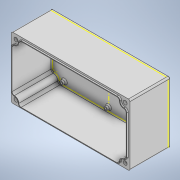
# Autodesk Inventor part: CustomBox_Rev3a
Saved by Autodesk Inventor 2021 (Build 250183000, 183)
## iProperties
Created: 2021-04-04
Part Number: CustomBox_Rev3a
Material: Generic
Document SubType Name: Modeling
Designer: James
Density: 1 g/cm^3
Appearance: Default
wall_thickness: 3.000 mm
lid_screw_d: 4.000 mm
lid_screw_offset_w: 3.182 mm
min_wall_width: 1.000 mm
inner_gasket_wall: 0.800 mm
inner_gasket_wall_h: 2.000 mm
pem_height: 4.000 mm
PEM_fillet: 1.500 mm
corner_fillet: 2.000 mm
inner_fillet: 1.000 mm
bottom_fillet: 1.000 mm
Author: James
Autodesk Inventor part; units mm, degrees
sketch "Sketch2" plane through (0, 0, 0) normal (0, 0, 1) x (1, 0, 0)
  line L0 (-78, 40.5) -> (78, 40.5)
  line L1 (78, 40.5) -> (78, -40.5)
  line L2 (78, -40.5) -> (-78, -40.5)
  line L3 (-78, -40.5) -> (-78, 40.5)
  line L4 (-78, 40.5) -> (78, -40.5) construction
  line L5 (78, 40.5) -> (-78, -40.5) construction
  line L6 (0, 40.5) -> (0, -40.5)
  line L7 (-78, 0) -> (78, 0)
  circle A0 centre (-71.818, 34.318) radius 2.5
  line L8 (-75, 29.545) -> (-67.045, 29.545) construction
  line L9 (-67.045, 29.545) -> (-67.045, 37.5) construction
  line L10 (75, 37.5) -> (-63.0835, 37.5) construction
  line L11 (-75, 25.5835) -> (-75, -37.5) construction
  line L12 (-75, -37.5) -> (75, -37.5) construction
  line L13 (75, -37.5) -> (75, 37.5) construction
  line L14 (-75, 37.5) -> (-67.045, 29.545) construction
  arc A1 (-71.9375, 28.5829) -> (-66.0829, 34.4375) centre (-71.818, 34.318) ccw
  arc A2 (-71.9375, 28.5829) -> (-75, 25.5835) centre (-72, 25.5835) ccw
  arc A3 (-63.0835, 37.5) -> (-66.0829, 34.4375) centre (-63.0835, 34.5) ccw
  line L15 (-75, 25.5835) -> (-75, 0)
  line L16 (-63.0835, 37.5) -> (0, 37.5)
  arc A4 (-66.0829, -34.4375) -> (-71.9375, -28.5829) centre (-71.818, -34.318) ccw
  arc A5 (-75, -25.5835) -> (-71.9375, -28.5829) centre (-72, -25.5835) ccw
  arc A6 (-66.0829, -34.4375) -> (-63.0835, -37.5) centre (-63.0835, -34.5) ccw
  line L17 (-75, -25.5835) -> (-75, 0)
  line L18 (-63.0835, -37.5) -> (0, -37.5)
  arc A7 (66.0829, 34.4375) -> (71.9375, 28.5829) centre (71.818, 34.318) ccw
  arc A8 (75, 25.5835) -> (71.9375, 28.5829) centre (72, 25.5835) ccw
  arc A9 (66.0829, 34.4375) -> (63.0835, 37.5) centre (63.0835, 34.5) ccw
  line L19 (75, 25.5835) -> (75, 0)
  line L20 (63.0835, 37.5) -> (0, 37.5)
  line L21 (63.0835, -37.5) -> (0, -37.5)
  arc A10 (63.0835, -37.5) -> (66.0829, -34.4375) centre (63.0835, -34.5) ccw
  arc A11 (71.9375, -28.5829) -> (66.0829, -34.4375) centre (71.818, -34.318) ccw
  arc A12 (71.9375, -28.5829) -> (75, -25.5835) centre (72, -25.5835) ccw
  line L22 (75, -25.5835) -> (75, 0)
  circle A13 centre (-71.818, -34.318) radius 2.5
  circle A14 centre (71.818, 34.318) radius 2.5
  circle A15 centre (71.818, -34.318) radius 2.5
  line L23 (0, 37.5) -> (-75, 37.5) construction
  line L24 (-75, 0) -> (-75, 37.5) construction
  point P0 (0, 0)
  point P1 (-75, 29.545)
  dimension "d5" = 156
  dimension "d6" = 81
  dimension "d11" = 5
  dimension "d23" = 3
  dimension "lid_screw_offset_w" = 3.182
  dimension "d26" = 7.955
  dimension "d27" = 7.955
  dimension "d28" = 3
  constraints: 50 end point, 26 point on circle, 26 symmetric about line, 16 centre point, 10 point on line, 6 midpoint, 4 parallel, 4 perpendicular, 4 tangent, 3 horizontal, 1 coincident, 1 equal radius, 15 other
  measures "d5" distance of L1.end L2.end
  measures "d6" distance of L0.end L1.end
  measures "d11" diameter of A0
  measures "d23" distance between parallel lines of L0 L10
  measures "lid_screw_offset_w" distance from line of A0.centre L11
  measures "d26" distance between parallel lines of L9 L11
  measures "d27" distance between parallel lines of L8 L10
  measures "d28" radius of A2
extrude "Extrusion1" add sketch "Sketch2" against normal blind 3 contours L0 L6 L16 A3 A1 A2 L15 L7 L3 | L0 L1 L7 L19 A8 A7 A9 L20 L6 | L7 L17 A5 A4 A6 L18 L6 L2 L3 | L20 A9 A7 A8 L19 L7 L6 | L6 L7 L15 A2 A1 A3 L16 | L7 L6 L18 A6 A4 A5 L17 | L1 L2 L6 L21 A10 A11 A12 L22 L7 | L7 L22 A12 A11 A10 L21 L6 | A0 | A13 | A14 | A15
extrude "Extrusion2" add sketch "Sketch2" along normal blind 50 contours L0 L6 L16 A3 A1 A2 L15 L7 L3 | L0 L1 L7 L19 A8 A7 A9 L20 L6 | L7 L17 A5 A4 A6 L18 L6 L2 L3 | L1 L2 L6 L21 A10 A11 A12 L22 L7
fillet "Fillet1" radius 2 4 edges at (-78, 40.5, 23.5) (-78, -40.5, 23.5) (78, -40.5, 23.5) (78, 40.5, 23.5)
fillet "Fillet2" radius 1 16 edges at (-65.2268, 36.5991, 0) (-67.7618, 30.2618, 0) (-74.0991, 27.7268, 0) (-75, 0, 0) (-74.0991, -27.7268, 0) (-67.7618, -30.2618, 0) (-65.2268, -36.5991, 0) (0, -37.5, 0) (65.2268, -36.5991, 0) (67.7618, -30.2618, 0) (74.0991, -27.7268, 0) (75, 0, 0) (74.0991, 27.7268, 0) (67.7618, 30.2618, 0) (65.2268, 36.5991, 0) (0, 37.5, 0)
fillet "Fillet3" radius 1 8 edges at (-77.4142, 39.9142, -3) (0, 40.5, -3) (77.4142, 39.9142, -3) (78, 0, -3) (77.4142, -39.9142, -3) (0, -40.5, -3) (-77.4142, -39.9142, -3) (-78, 0, -3)
ref_plane "Work Plane1" through (78, -40.5, 0) normal (0, 0, -1) x (-1, 0, 0)
sketch "Sketch3" plane through (78, -40.5, 0) normal (0, 0, -1) x (-1, 0, 0)
  line L0 (156, 79) -> (156, 2) projected
  line L1 (154, 0) -> (2, 0) projected
  line L2 (2, 81) -> (154, 81) projected
  line L3 (0, 2) -> (0, 79) projected
  line L4 (78, 81) -> (78, 0) projected
  line L5 (156, 40.5) -> (0, 40.5) projected
  line L6 (14.9165, 4) -> (141.0835, 4) projected
  line L7 (152, 14.9165) -> (152, 66.0835) projected
  line L8 (141.0835, 77) -> (14.9165, 77) projected
  line L9 (4, 66.0835) -> (4, 14.9165) projected
  arc A0 (12.9169, 6.0417) -> (6.0417, 12.9169) centre (6.182, 6.182) ccw projected
  arc A1 (6.0417, 68.0831) -> (12.9169, 74.9583) centre (6.182, 74.818) ccw projected
  arc A2 (143.0831, 74.9583) -> (149.9583, 68.0831) centre (149.818, 74.818) ccw projected
  arc A3 (149.9583, 12.9169) -> (143.0831, 6.0417) centre (149.818, 6.182) ccw projected
  circle A4 centre (136.0835, 9) radius 1.25
  circle A5 centre (136.0835, 9) radius 2.25
  circle A6 centre (136.0835, 72) radius 1.25
  circle A7 centre (136.0835, 72) radius 2.25
  circle A8 centre (19.9165, 9) radius 1.25
  circle A9 centre (19.9165, 9) radius 2.25
  circle A10 centre (19.9165, 72) radius 1.25
  circle A11 centre (19.9165, 72) radius 2.25
  circle A12 centre (147, 40.5) radius 1.25
  circle A13 centre (147, 40.5) radius 2.25
  circle A14 centre (9, 40.5) radius 1.25
  circle A15 centre (9, 40.5) radius 2.25
  circle A16 centre (78, 9) radius 1.25
  circle A17 centre (78, 9) radius 2.25
  circle A18 centre (78, 72) radius 1.25
  circle A19 centre (78, 72) radius 2.25
  point P0 (78, 40.5)
  point P1 (14.9165, 6)
  point P2 (6, 14.9165)
  point P3 (6, 66.0835)
  point P4 (14.9165, 75)
  point P5 (141.0835, 75)
  point P6 (150, 66.0835)
  point P7 (150, 14.9165)
  point P8 (141.0835, 6)
  dimension "mounting_hole_d" = 2.5
  dimension "d37" = 4.5
  dimension "d38" = 5
  dimension "d39" = 5
  dimension "d40" = 2.5
  dimension "d41" = 4.5
  dimension "mounting_hole_offset" = 5
  dimension "d43" = 2.5
  dimension "d44" = 4.5
  dimension "d45" = 5
  constraints: 16 centre point, 10 symmetric about line, 8 coincident, 2 point on line, 10 other
  measures "mounting_hole_d" diameter of A4
  measures "d37" diameter of A5
  measures "d38" distance from line of L6 A4.centre
  measures "d39" horizontal distance of L6.end A4.centre
  measures "d40" diameter of A12
  measures "d41" diameter of A13
  measures "mounting_hole_offset" distance from line of L7 A12.centre
  measures "d43" diameter of A16
  measures "d44" diameter of A17
  measures "d45" distance from line of L6 A16.centre
extrude "Extrusion3" add sketch "Sketch3" against normal blind 4 contours A19 L4 A18 | L4 A18 A19 | A18 L4 | L4 A18 | A17 L4 A16 | L4 A16 A17 | A16 L4 | L4 A16 | A13 L5 A12 | L5 A12 A13 | A12 L5 | L5 A12 | A15 L5 A14 | L5 A14 A15 | A14 L5 | L5 A14 | A4 | A5 | A6 | A7 | A8 | A9 | A10 | A11
extrude "Extrusion4" cut sketch "Sketch3" against normal blind 4 contours A18 L4 | L4 A18 | A16 L4 | L4 A16 | A12 L5 | L5 A12 | A14 L5 | L5 A14 | A4 | A6 | A8 | A10
fillet "Fillet4" radius 1.5 8 edges at (-55.8335, -31.5, 0) (-66.75, 0, 0) (2.25, -31.5, 0) (60.3335, -31.5, 0) (-55.8335, 31.5, 0) (2.25, 31.5, 0) (60.3335, 31.5, 0) (71.25, 0, 0)
sketch "Sketch4" plane through (0, 0, 50) normal (0, 0, 1) x (1, 0, 0)
  line L0 (75, 25.5835) -> (75, -25.5835) projected
  arc A0 (71.9375, -28.5829) -> (75, -25.5835) centre (72, -25.5835) ccw projected
  arc A1 (71.9375, -28.5829) -> (66.0829, -34.4375) centre (71.818, -34.318) ccw projected
  arc A2 (63.0835, -37.5) -> (66.0829, -34.4375) centre (63.0835, -34.5) ccw projected
  line L1 (63.0835, -37.5) -> (-63.0835, -37.5) projected
  arc A3 (-66.0829, -34.4375) -> (-63.0835, -37.5) centre (-63.0835, -34.5) ccw projected
  arc A4 (-66.0829, -34.4375) -> (-71.9375, -28.5829) centre (-71.818, -34.318) ccw projected
  arc A5 (-75, -25.5835) -> (-71.9375, -28.5829) centre (-72, -25.5835) ccw projected
  line L2 (-75, -25.5835) -> (-75, 25.5835) projected
  arc A6 (-71.9375, 28.5829) -> (-75, 25.5835) centre (-72, 25.5835) ccw projected
  arc A7 (-71.9375, 28.5829) -> (-66.0829, 34.4375) centre (-71.818, 34.318) ccw projected
  arc A8 (-63.0835, 37.5) -> (-66.0829, 34.4375) centre (-63.0835, 34.5) ccw projected
  line L3 (-63.0835, 37.5) -> (63.0835, 37.5) projected
  arc A9 (66.0829, 34.4375) -> (63.0835, 37.5) centre (63.0835, 34.5) ccw projected
  arc A10 (66.0829, 34.4375) -> (71.9375, 28.5829) centre (71.818, 34.318) ccw projected
  arc A11 (75, 25.5835) -> (71.9375, 28.5829) centre (72, 25.5835) ccw projected
  line L4 (63.0835, 38.3) -> (-63.0835, 38.3)
  arc A12 (-63.0835, 38.3) -> (-66.8827, 34.4208) centre (-63.0835, 34.5) ccw
  arc A13 (-71.9208, 29.3827) -> (-66.8827, 34.4208) centre (-71.818, 34.318) ccw
  arc A14 (-71.9208, 29.3827) -> (-75.8, 25.5835) centre (-72, 25.5835) ccw
  line L5 (-75.8, 25.5835) -> (-75.8, -25.5835)
  arc A15 (-75.8, -25.5835) -> (-71.9208, -29.3827) centre (-72, -25.5835) ccw
  arc A16 (-66.8827, -34.4208) -> (-71.9208, -29.3827) centre (-71.818, -34.318) ccw
  arc A17 (-66.8827, -34.4208) -> (-63.0835, -38.3) centre (-63.0835, -34.5) ccw
  line L6 (-63.0835, -38.3) -> (63.0835, -38.3)
  arc A18 (63.0835, -38.3) -> (66.8827, -34.4208) centre (63.0835, -34.5) ccw
  arc A19 (71.9208, -29.3827) -> (66.8827, -34.4208) centre (71.818, -34.318) ccw
  arc A20 (71.9208, -29.3827) -> (75.8, -25.5835) centre (72, -25.5835) ccw
  line L7 (75.8, -25.5835) -> (75.8, 25.5835)
  arc A21 (75.8, 25.5835) -> (71.9208, 29.3827) centre (72, 25.5835) ccw
  arc A22 (66.8827, 34.4208) -> (71.9208, 29.3827) centre (71.818, 34.318) ccw
  arc A23 (66.8827, 34.4208) -> (63.0835, 38.3) centre (63.0835, 34.5) ccw
  point P0 (0, 0)
  dimension "inner_gasket_wall" = 0.8
  constraints: 24 point on circle, 12 centre point, 8 end point, 15 other
  measures "inner_gasket_wall" distance between parallel lines of L3 L4
extrude "Extrusion5" add sketch "Sketch4" along normal blind 2
ref_plane "Inspection Plane" through (-69, 0, 0) normal (0, 1, 0) x (1, 0, 0)
sketch "Sketch5" plane through (-69, 0, 0) normal (0, 1, 0) x (1, 0, 0)
  point P0 (69, 0)
ref_plane "Floor" through (-63.0835, 36.5, 0) normal (0, 0, 1) x (1, 0, 0)
sketch "Sketch6" plane through (-63.0835, 36.5, 0) normal (0, 0, 1) x (1, 0, 0)
  line L0 (11.0727, -3.3545) -> (56.3334, -3.3545) construction
  line L1 (56.3334, -3.3545) -> (56.3334, -12.559) construction
  line L2 (56.3334, -12.559) -> (11.0727, -12.559) construction
  line L3 (11.0727, -12.559) -> (11.0727, -3.3545) construction
  line L4 (11.0528, -6.484) -> (12.0115, -4.9267)
  line L5 (12.0115, -4.9267) -> (11.0528, -3.434)
  line L6 (11.0528, -3.434) -> (11.778, -3.434)
  line L7 (11.778, -3.434) -> (12.4014, -4.4995)
  line L8 (12.4014, -4.4995) -> (13.0199, -3.434)
  line L9 (13.0199, -3.434) -> (13.7501, -3.434)
  line L10 (13.7501, -3.434) -> (12.7914, -4.9217)
  line L11 (12.7914, -4.9217) -> (13.7501, -6.484)
  line L12 (13.7501, -6.484) -> (13.0249, -6.484)
  line L13 (13.0249, -6.484) -> (12.4014, -5.4284)
  line L14 (12.4014, -5.4284) -> (11.778, -6.484)
  line L15 (11.778, -6.484) -> (11.0528, -6.484)
  line L16 (14.0432, -6.484) -> (14.0432, -3.434)
  line L17 (14.0432, -3.434) -> (16.2587, -3.434)
  line L18 (16.2587, -3.434) -> (16.2587, -3.9655)
  line L19 (16.2587, -3.9655) -> (14.6616, -3.9655)
  line L20 (14.6616, -3.9655) -> (14.6616, -4.6162)
  line L21 (14.6616, -4.6162) -> (16.122, -4.6162)
  line L22 (16.122, -4.6162) -> (16.122, -5.1378)
  line L23 (16.122, -5.1378) -> (14.6616, -5.1378)
  line L24 (14.6616, -5.1378) -> (14.6616, -5.9202)
  line L25 (14.6616, -5.9202) -> (16.3332, -5.9202)
  line L26 (16.3332, -5.9202) -> (16.3332, -6.484)
  line L27 (16.3332, -6.484) -> (14.0432, -6.484)
  spline S0 degree 2 poles (19.4676, -5.4358) (19.4328, -5.9549) (18.7001, -6.5684) (18.114, -6.5684) knots 0 0 0 1 2 2 2
  spline S1 degree 2 poles (18.114, -6.5684) (17.4359, -6.5684) (16.6834, -5.7239) (16.6834, -4.9614) knots 0 0 0 1 2 2 2
  spline S2 degree 2 poles (16.6834, -4.9614) (16.6834, -4.1816) (17.4508, -3.3545) (18.1686, -3.3545) knots 0 0 0 1 2 2 2
  spline S3 degree 2 poles (18.1686, -3.3545) (18.7523, -3.3545) (19.4304, -3.9257) (19.4626, -4.4448) knots 0 0 0 1 2 2 2
  line L28 (19.4626, -4.4448) -> (18.8442, -4.4448)
  spline S4 degree 2 poles (18.8442, -4.4448) (18.8045, -4.184) (18.4617, -3.9133) (18.1686, -3.9133) knots 0 0 0 1 2 2 2
  spline S5 degree 2 poles (18.1686, -3.9133) (17.7538, -3.9133) (17.3242, -4.4473) (17.3242, -4.9614) knots 0 0 0 1 2 2 2
  spline S6 degree 2 poles (17.3242, -4.9614) (17.3242, -5.4582) (17.7538, -5.9996) (18.1488, -5.9996) knots 0 0 0 1 2 2 2
  spline S7 degree 2 poles (18.1488, -5.9996) (18.4344, -5.9996) (18.797, -5.709) (18.8517, -5.4358) knots 0 0 0 1 2 2 2
  line L29 (18.8517, -5.4358) -> (19.4676, -5.4358)
  line L30 (19.9495, -3.424) -> (20.5828, -3.424)
  line L31 (20.5828, -3.424) -> (20.5828, -5.3365)
  spline S8 degree 2 poles (20.5828, -5.3365) (20.5828, -5.6916) (20.8635, -6.017) (21.1714, -6.017) knots 0 0 0 1 2 2 2
  spline S9 degree 2 poles (21.1714, -6.017) (21.4819, -6.017) (21.765, -5.6941) (21.765, -5.3365) knots 0 0 0 1 2 2 2
  line L32 (21.765, -5.3365) -> (21.765, -3.424)
  line L33 (21.765, -3.424) -> (22.3934, -3.424)
  line L34 (22.3934, -3.424) -> (22.3934, -5.406)
  spline S10 degree 2 poles (22.3934, -5.406) (22.3934, -5.9673) (21.765, -6.5684) (21.1764, -6.5684) knots 0 0 0 1 2 2 2
  spline S11 degree 2 poles (21.1764, -6.5684) (20.5803, -6.5684) (19.9495, -5.9698) (19.9495, -5.406) knots 0 0 0 1 2 2 2
  line L35 (19.9495, -5.406) -> (19.9495, -3.424)
  line L36 (23.6427, -6.484) -> (23.6427, -3.9779)
  line L37 (23.6427, -3.9779) -> (22.7387, -3.9779)
  line L38 (22.7387, -3.9779) -> (22.7387, -3.434)
  line L39 (22.7387, -3.434) -> (25.1702, -3.434)
  line L40 (25.1702, -3.434) -> (25.1702, -3.9779)
  line L41 (25.1702, -3.9779) -> (24.2711, -3.9779)
  line L42 (24.2711, -3.9779) -> (24.2711, -6.484)
  line L43 (24.2711, -6.484) -> (23.6427, -6.484)
  line L44 (25.5328, -6.484) -> (25.5328, -3.434)
  line L45 (25.5328, -3.434) -> (27.7483, -3.434)
  line L46 (27.7483, -3.434) -> (27.7483, -3.9655)
  line L47 (27.7483, -3.9655) -> (26.1513, -3.9655)
  line L48 (26.1513, -3.9655) -> (26.1513, -4.6162)
  line L49 (26.1513, -4.6162) -> (27.6117, -4.6162)
  line L50 (27.6117, -4.6162) -> (27.6117, -5.1378)
  line L51 (27.6117, -5.1378) -> (26.1513, -5.1378)
  line L52 (26.1513, -5.1378) -> (26.1513, -5.9202)
  line L53 (26.1513, -5.9202) -> (27.8228, -5.9202)
  line L54 (27.8228, -5.9202) -> (27.8228, -6.484)
  line L55 (27.8228, -6.484) -> (25.5328, -6.484)
  line L56 (30.2271, -6.484) -> (29.174, -3.434)
  line L57 (29.174, -3.434) -> (29.8694, -3.434)
  line L58 (29.8694, -3.434) -> (30.5201, -5.7165)
  line L59 (30.5201, -5.7165) -> (31.1808, -3.434)
  line L60 (31.1808, -3.434) -> (31.8688, -3.434)
  line L61 (31.8688, -3.434) -> (30.8281, -6.484)
  line L62 (30.8281, -6.484) -> (30.2271, -6.484)
  line L63 (33.4956, -5.8009) -> (34.0967, -5.8009)
  spline S12 degree 2 poles (34.0967, -5.8009) (34.0048, -6.1561) (33.4534, -6.5609) (33.056, -6.5609) knots 0 0 0 1 2 2 2
  spline S13 degree 2 poles (33.056, -6.5609) (32.5667, -6.5609) (31.9955, -5.9052) (31.9955, -5.3439) knots 0 0 0 1 2 2 2
  spline S14 degree 2 poles (31.9955, -5.3439) (31.9955, -4.7901) (32.5593, -4.1517) (33.0486, -4.1517) knots 0 0 0 1 2 2 2
  spline S15 degree 2 poles (33.0486, -4.1517) (33.5652, -4.1517) (34.129, -4.7801) (34.129, -5.3613) knots 0 0 0 1 2 2 2
  spline S16 degree 2 poles (34.129, -5.3613) (34.129, -5.4234) (34.1265, -5.488) (34.1215, -5.5178) knots 0 0 0 1 2 2 2
  line L64 (34.1215, -5.5178) -> (32.6189, -5.5178)
  spline S17 degree 2 poles (32.6189, -5.5178) (32.6313, -5.7835) (32.8648, -6.0518) (33.0833, -6.0518) knots 0 0 0 1 2 2 2
  spline S18 degree 2 poles (33.0833, -6.0518) (33.2398, -6.0518) (33.4385, -5.9301) (33.4956, -5.8009) knots 0 0 0 1 2 2 2
  line L65 (32.6189, -5.1229) -> (33.5056, -5.1229)
  spline S19 degree 2 poles (33.5056, -5.1229) (33.4981, -4.8944) (33.2721, -4.6559) (33.061, -4.6559) knots 0 0 0 1 2 2 2
  spline S20 degree 2 poles (33.061, -4.6559) (32.8623, -4.6559) (32.6387, -4.8969) (32.6189, -5.1229) knots 0 0 0 1 2 2 2
  line L66 (34.5288, -6.484) -> (34.5288, -4.2312)
  line L67 (34.5288, -4.2312) -> (35.12, -4.2312)
  line L68 (35.12, -4.2312) -> (35.12, -4.4995)
  spline S21 degree 2 poles (35.12, -4.4995) (35.2466, -4.3355) (35.5894, -4.1716) (35.8005, -4.1716) knots 0 0 0 1 2 2 2
  spline S22 degree 2 poles (35.8005, -4.1716) (36.1731, -4.1716) (36.5431, -4.5591) (36.5431, -4.949) knots 0 0 0 1 2 2 2
  line L69 (36.5431, -4.949) -> (36.5431, -6.484)
  line L70 (36.5431, -6.484) -> (35.9396, -6.484)
  line L71 (35.9396, -6.484) -> (35.9396, -5.1229)
  spline S23 degree 2 poles (35.9396, -5.1229) (35.9396, -4.8795) (35.7757, -4.6733) (35.5919, -4.6733) knots 0 0 0 1 2 2 2
  spline S24 degree 2 poles (35.5919, -4.6733) (35.3808, -4.6733) (35.1324, -4.9291) (35.1324, -5.1477) knots 0 0 0 1 2 2 2
  line L72 (35.1324, -5.1477) -> (35.1324, -6.484)
  line L73 (35.1324, -6.484) -> (34.5288, -6.484)
  spline S25 degree 2 poles (38.0607, -6.5013) (37.9787, -6.5038) (37.7477, -6.5138) (37.7179, -6.5138) knots 0 0 0 1 2 2 2
  spline S26 degree 2 poles (37.7179, -6.5138) (37.3727, -6.5138) (37.1169, -6.2555) (37.1169, -5.873) knots 0 0 0 1 2 2 2
  line L74 (37.1169, -5.873) -> (37.1169, -4.6535)
  line L75 (37.1169, -4.6535) -> (36.8188, -4.6535)
  line L76 (36.8188, -4.6535) -> (36.8188, -4.2312)
  line L77 (36.8188, -4.2312) -> (37.1169, -4.2312)
  line L78 (37.1169, -4.2312) -> (37.1169, -3.6177)
  line L79 (37.1169, -3.6177) -> (37.713, -3.6177)
  line L80 (37.713, -3.6177) -> (37.713, -4.2312)
  line L81 (37.713, -4.2312) -> (38.0607, -4.2312)
  line L82 (38.0607, -4.2312) -> (38.0607, -4.6535)
  line L83 (38.0607, -4.6535) -> (37.713, -4.6535)
  line L84 (37.713, -4.6535) -> (37.713, -5.9028)
  spline S27 degree 2 poles (37.713, -5.9028) (37.713, -5.9897) (37.7924, -6.0468) (37.9142, -6.0468) knots 0 0 0 1 2 2 2
  line L85 (37.9142, -6.0468) -> (38.0607, -6.0468)
  line L86 (38.0607, -6.0468) -> (38.0607, -6.5013)
  line L87 (40.4177, -4.2312) -> (40.4177, -6.484)
  line L88 (40.4177, -6.484) -> (39.8266, -6.484)
  line L89 (39.8266, -6.484) -> (39.8266, -6.2157)
  spline S28 degree 2 poles (39.8266, -6.2157) (39.6975, -6.3796) (39.3572, -6.5436) (39.1436, -6.5436) knots 0 0 0 1 2 2 2
  spline S29 degree 2 poles (39.1436, -6.5436) (38.7735, -6.5436) (38.4034, -6.1536) (38.4034, -5.7662) knots 0 0 0 1 2 2 2
  line L90 (38.4034, -5.7662) -> (38.4034, -4.2312)
  line L91 (38.4034, -4.2312) -> (39.007, -4.2312)
  line L92 (39.007, -4.2312) -> (39.007, -5.5923)
  spline S30 degree 2 poles (39.007, -5.5923) (39.007, -5.8307) (39.1684, -6.0369) (39.3547, -6.0369) knots 0 0 0 1 2 2 2
  spline S31 degree 2 poles (39.3547, -6.0369) (39.5633, -6.0369) (39.8142, -5.7811) (39.8142, -5.5625) knots 0 0 0 1 2 2 2
  line L93 (39.8142, -5.5625) -> (39.8142, -4.2312)
  line L94 (39.8142, -4.2312) -> (40.4177, -4.2312)
  line L95 (40.9443, -6.484) -> (40.9443, -4.2312)
  line L96 (40.9443, -4.2312) -> (41.5031, -4.2312)
  line L97 (41.5031, -4.2312) -> (41.5031, -4.6187)
  spline S32 degree 2 poles (41.5031, -4.6187) (41.6223, -4.3877) (41.9378, -4.1691) (42.1538, -4.1691) knots 0 0 0 1 2 2 2
  spline S33 degree 2 poles (42.1538, -4.1691) (42.1886, -4.1691) (42.2284, -4.1716) (42.2408, -4.1741) knots 0 0 0 1 2 2 2
  line L98 (42.2408, -4.1741) -> (42.2433, -4.7851)
  line L99 (42.2433, -4.7851) -> (42.0421, -4.7851)
  spline S34 degree 2 poles (42.0421, -4.7851) (41.7962, -4.7851) (41.5478, -5.0409) (41.5478, -5.2943) knots 0 0 0 1 2 2 2
  line L100 (41.5478, -5.2943) -> (41.5478, -6.484)
  line L101 (41.5478, -6.484) -> (40.9443, -6.484)
  line L102 (43.9595, -5.8009) -> (44.5606, -5.8009)
  spline S35 degree 2 poles (44.5606, -5.8009) (44.4687, -6.1561) (43.9173, -6.5609) (43.5199, -6.5609) knots 0 0 0 1 2 2 2
  spline S36 degree 2 poles (43.5199, -6.5609) (43.0306, -6.5609) (42.4593, -5.9052) (42.4593, -5.3439) knots 0 0 0 1 2 2 2
  spline S37 degree 2 poles (42.4593, -5.3439) (42.4593, -4.7901) (43.0231, -4.1517) (43.5124, -4.1517) knots 0 0 0 1 2 2 2
  spline S38 degree 2 poles (43.5124, -4.1517) (44.0291, -4.1517) (44.5929, -4.7801) (44.5929, -5.3613) knots 0 0 0 1 2 2 2
  spline S39 degree 2 poles (44.5929, -5.3613) (44.5929, -5.4234) (44.5904, -5.488) (44.5854, -5.5178) knots 0 0 0 1 2 2 2
  line L103 (44.5854, -5.5178) -> (43.0828, -5.5178)
  spline S40 degree 2 poles (43.0828, -5.5178) (43.0952, -5.7835) (43.3286, -6.0518) (43.5472, -6.0518) knots 0 0 0 1 2 2 2
  spline S41 degree 2 poles (43.5472, -6.0518) (43.7037, -6.0518) (43.9024, -5.9301) (43.9595, -5.8009) knots 0 0 0 1 2 2 2
  line L104 (43.0828, -5.1229) -> (43.9694, -5.1229)
  spline S42 degree 2 poles (43.9694, -5.1229) (43.962, -4.8944) (43.736, -4.6559) (43.5249, -4.6559) knots 0 0 0 1 2 2 2
  spline S43 degree 2 poles (43.5249, -4.6559) (43.3262, -4.6559) (43.1026, -4.8969) (43.0828, -5.1229) knots 0 0 0 1 2 2 2
  line L105 (44.8661, -5.7513) -> (45.4671, -5.7513)
  spline S44 degree 2 poles (45.4671, -5.7513) (45.4746, -5.9226) (45.708, -6.0915) (45.939, -6.0915) knots 0 0 0 1 2 2 2
  spline S45 degree 2 poles (45.939, -6.0915) (46.1154, -6.0915) (46.3091, -5.9723) (46.3091, -5.8655) knots 0 0 0 1 2 2 2
  spline S46 degree 2 poles (46.3091, -5.8655) (46.3091, -5.7115) (45.949, -5.6345) knots 0 0 0 1 1 1
  spline S47 degree 2 poles (45.949, -5.6345) (45.8024, -5.6047) (45.7155, -5.5824) knots 0 0 0 1 1 1
  spline S48 degree 2 poles (45.7155, -5.5824) (45.2759, -5.4706) (44.9331, -5.1626) (44.9331, -4.9018) knots 0 0 0 1 2 2 2
  spline S49 degree 2 poles (44.9331, -4.9018) (44.9331, -4.5566) (45.4324, -4.1517) (45.8596, -4.1517) knots 0 0 0 1 2 2 2
  spline S50 degree 2 poles (45.8596, -4.1517) (46.3116, -4.1517) (46.8257, -4.5541) (46.8431, -4.9192) knots 0 0 0 1 2 2 2
  line L106 (46.8431, -4.9192) -> (46.2569, -4.9192)
  spline S51 degree 2 poles (46.2569, -4.9192) (46.252, -4.7752) (46.0458, -4.6187) (45.8645, -4.6187) knots 0 0 0 1 2 2 2
  spline S52 degree 2 poles (45.8645, -4.6187) (45.6931, -4.6187) (45.5242, -4.723) (45.5242, -4.8248) knots 0 0 0 1 2 2 2
  spline S53 degree 2 poles (45.5242, -4.8248) (45.5242, -4.9614) (45.9738, -5.0633) knots 0 0 0 1 1 1
  spline S54 degree 2 poles (45.9738, -5.0633) (46.0781, -5.0856) (46.1377, -5.1005) knots 0 0 0 1 1 1
  spline S55 degree 2 poles (46.1377, -5.1005) (46.5873, -5.2073) (46.9151, -5.5054) (46.9151, -5.7761) knots 0 0 0 1 2 2 2
  spline S56 degree 2 poles (46.9151, -5.7761) (46.9151, -6.1586) (46.3737, -6.5609) (45.8596, -6.5609) knots 0 0 0 1 2 2 2
  spline S57 degree 2 poles (45.8596, -6.5609) (45.3926, -6.5609) (44.8661, -6.1437) (44.8661, -5.7761) knots 0 0 0 1 2 2 2
  line L107 (44.8661, -5.7761) -> (44.8661, -5.7513)
  line L108 (48.5693, -6.484) -> (48.5693, -3.434)
  line L109 (48.5693, -3.434) -> (49.1977, -3.434)
  line L110 (49.1977, -3.434) -> (49.1977, -5.9202)
  line L111 (49.1977, -5.9202) -> (50.6854, -5.9202)
  line L112 (50.6854, -5.9202) -> (50.6854, -6.484)
  line L113 (50.6854, -6.484) -> (48.5693, -6.484)
  line L114 (51.0306, -6.484) -> (51.0306, -3.434)
  line L115 (51.0306, -3.434) -> (51.659, -3.434)
  line L116 (51.659, -3.434) -> (51.659, -5.9202)
  line L117 (51.659, -5.9202) -> (53.1468, -5.9202)
  line L118 (53.1468, -5.9202) -> (53.1468, -6.484)
  line L119 (53.1468, -6.484) -> (51.0306, -6.484)
  spline S58 degree 2 poles (56.1471, -5.4358) (56.1123, -5.9549) (55.3796, -6.5684) (54.7935, -6.5684) knots 0 0 0 1 2 2 2
  spline S59 degree 2 poles (54.7935, -6.5684) (54.1154, -6.5684) (53.3628, -5.7239) (53.3628, -4.9614) knots 0 0 0 1 2 2 2
  spline S60 degree 2 poles (53.3628, -4.9614) (53.3628, -4.1816) (54.1303, -3.3545) (54.8481, -3.3545) knots 0 0 0 1 2 2 2
  spline S61 degree 2 poles (54.8481, -3.3545) (55.4318, -3.3545) (56.1098, -3.9257) (56.1421, -4.4448) knots 0 0 0 1 2 2 2
  line L120 (56.1421, -4.4448) -> (55.5237, -4.4448)
  spline S62 degree 2 poles (55.5237, -4.4448) (55.4839, -4.184) (55.1412, -3.9133) (54.8481, -3.9133) knots 0 0 0 1 2 2 2
  spline S63 degree 2 poles (54.8481, -3.9133) (54.4333, -3.9133) (54.0036, -4.4473) (54.0036, -4.9614) knots 0 0 0 1 2 2 2
  spline S64 degree 2 poles (54.0036, -4.9614) (54.0036, -5.4582) (54.4333, -5.9996) (54.8282, -5.9996) knots 0 0 0 1 2 2 2
  spline S65 degree 2 poles (54.8282, -5.9996) (55.1139, -5.9996) (55.4765, -5.709) (55.5311, -5.4358) knots 0 0 0 1 2 2 2
  line L121 (55.5311, -5.4358) -> (56.1471, -5.4358)
  line L122 (11.3484, -12.559) -> (11.3484, -9.4022)
  line L123 (11.3484, -9.4022) -> (11.9221, -9.4022)
  line L124 (11.9221, -9.4022) -> (11.9221, -9.7102)
  spline S66 degree 2 poles (11.9221, -9.7102) (12.0537, -9.509) (12.3741, -9.3277) (12.5927, -9.3277) knots 0 0 0 1 2 2 2
  spline S67 degree 2 poles (12.5927, -9.3277) (13.0075, -9.3277) (13.5266, -9.9834) (13.5266, -10.5174) knots 0 0 0 1 2 2 2
  spline S68 degree 2 poles (13.5266, -10.5174) (13.5266, -11.0588) (13.0075, -11.7319) (12.6001, -11.7319) knots 0 0 0 1 2 2 2
  spline S69 degree 2 poles (12.6001, -11.7319) (12.3841, -11.7319) (12.0463, -11.5506) (11.9345, -11.3768) knots 0 0 0 1 2 2 2
  line L125 (11.9345, -11.3768) -> (11.9345, -12.559)
  line L126 (11.9345, -12.559) -> (11.3484, -12.559)
  spline S70 degree 2 poles (12.928, -10.5447) (12.928, -10.2044) (12.6697, -9.8468) (12.4263, -9.8468) knots 0 0 0 1 2 2 2
  spline S71 degree 2 poles (12.4263, -9.8468) (12.1854, -9.8468) (11.9345, -10.202) (11.9345, -10.5447) knots 0 0 0 1 2 2 2
  spline S72 degree 2 poles (11.9345, -10.5447) (11.9345, -10.8626) (12.1978, -11.2103) (12.4387, -11.2103) knots 0 0 0 1 2 2 2
  spline S73 degree 2 poles (12.4387, -11.2103) (12.6672, -11.2103) (12.928, -10.8552) (12.928, -10.5447) knots 0 0 0 1 2 2 2
  line L127 (13.6905, -12.0498) -> (14.7188, -8.5255)
  line L128 (14.7188, -8.5255) -> (15.0019, -8.5255)
  line L129 (15.0019, -8.5255) -> (13.9712, -12.0498)
  line L130 (13.9712, -12.0498) -> (13.6905, -12.0498)
  line L131 (15.2801, -11.6549) -> (15.2801, -9.4022)
  line L132 (15.2801, -9.4022) -> (15.8712, -9.4022)
  line L133 (15.8712, -9.4022) -> (15.8712, -9.6704)
  spline S74 degree 2 poles (15.8712, -9.6704) (15.9979, -9.5065) (16.3406, -9.3426) (16.5517, -9.3426) knots 0 0 0 1 2 2 2
  spline S75 degree 2 poles (16.5517, -9.3426) (16.9243, -9.3426) (17.2944, -9.7301) (17.2944, -10.12) knots 0 0 0 1 2 2 2
  line L134 (17.2944, -10.12) -> (17.2944, -11.6549)
  line L135 (17.2944, -11.6549) -> (16.6908, -11.6549)
  line L136 (16.6908, -11.6549) -> (16.6908, -10.2939)
  spline S76 degree 2 poles (16.6908, -10.2939) (16.6908, -10.0505) (16.5269, -9.8443) (16.3431, -9.8443) knots 0 0 0 1 2 2 2
  spline S77 degree 2 poles (16.3431, -9.8443) (16.132, -9.8443) (15.8836, -10.1001) (15.8836, -10.3187) knots 0 0 0 1 2 2 2
  line L137 (15.8836, -10.3187) -> (15.8836, -11.6549)
  line L138 (15.8836, -11.6549) -> (15.2801, -11.6549)
  spline S78 degree 2 poles (18.8566, -11.6549) (18.8616, -11.2575) (19.1919, -10.7037) (19.6142, -10.4205) knots 0 0 0 1 2 2 2
  spline S79 degree 2 poles (19.6142, -10.4205) (19.6787, -10.3758) (19.8004, -10.3013) knots 0 0 0 1 1 1
  spline S80 degree 2 poles (19.8004, -10.3013) (20.3593, -9.9412) (20.3593, -9.6108) knots 0 0 0 1 1 1
  spline S81 degree 2 poles (20.3593, -9.6108) (20.3593, -9.4146) (20.1233, -9.1861) (19.9196, -9.1861) knots 0 0 0 1 2 2 2
  spline S82 degree 2 poles (19.9196, -9.1861) (19.6961, -9.1861) (19.4527, -9.4668) (19.4527, -9.7251) knots 0 0 0 1 2 2 2
  line L139 (19.4527, -9.7251) -> (19.4527, -9.7499)
  line L140 (19.4527, -9.7499) -> (18.9063, -9.7499)
  spline S83 degree 2 poles (18.9063, -9.7499) (18.9063, -9.2408) (19.4527, -8.6894) (19.9594, -8.6894) knots 0 0 0 1 2 2 2
  spline S84 degree 2 poles (19.9594, -8.6894) (20.4164, -8.6894) (20.9628, -9.1886) (20.9628, -9.6009) knots 0 0 0 1 2 2 2
  spline S85 degree 2 poles (20.9628, -9.6009) (20.9628, -9.8989) (20.6772, -10.3336) (20.2674, -10.6093) knots 0 0 0 1 2 2 2
  spline S86 degree 2 poles (20.2674, -10.6093) (20.1804, -10.6689) (20.0264, -10.7682) knots 0 0 0 1 1 1
  spline S87 degree 2 poles (20.0264, -10.7682) (19.6365, -11.0166) (19.5868, -11.1483) knots 0 0 0 1 1 1
  line L141 (19.5868, -11.1483) -> (20.933, -11.1483)
  line L142 (20.933, -11.1483) -> (20.933, -11.6549)
  line L143 (20.933, -11.6549) -> (18.8566, -11.6549)
  line L144 (22.5102, -11.6549) -> (22.5102, -11.0141)
  line L145 (22.5102, -11.0141) -> (21.2609, -11.0141)
  line L146 (21.2609, -11.0141) -> (21.2609, -10.4926)
  line L147 (21.2609, -10.4926) -> (22.3537, -8.7738)
  line L148 (22.3537, -8.7738) -> (23.0889, -8.7738)
  line L149 (23.0889, -8.7738) -> (23.0889, -10.5422)
  line L150 (23.0889, -10.5422) -> (23.4341, -10.5422)
  line L151 (23.4341, -10.5422) -> (23.4341, -11.0141)
  line L152 (23.4341, -11.0141) -> (23.0889, -11.0141)
  line L153 (23.0889, -11.0141) -> (23.0889, -11.6549)
  line L154 (23.0889, -11.6549) -> (22.5102, -11.6549)
  line L155 (22.5226, -10.5571) -> (22.5226, -9.288)
  line L156 (22.5226, -9.288) -> (21.7179, -10.5571)
  line L157 (21.7179, -10.5571) -> (22.5226, -10.5571)
  line L158 (24.6139, -11.6549) -> (24.6139, -9.6282)
  line L159 (24.6139, -9.6282) -> (23.906, -9.6282)
  line L160 (23.906, -9.6282) -> (23.906, -9.211)
  line L161 (23.906, -9.211) -> (23.9507, -9.211)
  spline S88 degree 2 poles (23.9507, -9.211) (24.3382, -9.211) (24.6933, -8.97) (24.7231, -8.6894) knots 0 0 0 1 2 2 2
  line L162 (24.7231, -8.6894) -> (25.1975, -8.6894)
  line L163 (25.1975, -8.6894) -> (25.1975, -11.6549)
  line L164 (25.1975, -11.6549) -> (24.6139, -11.6549)
  line L165 (26.1041, -10.8105) -> (26.1041, -10.2417)
  line L166 (26.1041, -10.2417) -> (27.269, -10.2417)
  line L167 (27.269, -10.2417) -> (27.269, -10.8105)
  line L168 (27.269, -10.8105) -> (26.1041, -10.8105)
  spline S89 degree 2 poles (27.5273, -10.2144) (27.5273, -9.4494) (28.0588, -8.6894) (28.5977, -8.6894) knots 0 0 0 1 2 2 2
  spline S90 degree 2 poles (28.5977, -8.6894) (29.1342, -8.6894) (29.6707, -9.4544) (29.6707, -10.2193) knots 0 0 0 1 2 2 2
  spline S91 degree 2 poles (29.6707, -10.2193) (29.6707, -10.9818) (29.1392, -11.7369) (28.5977, -11.7369) knots 0 0 0 1 2 2 2
  spline S92 degree 2 poles (28.5977, -11.7369) (28.0588, -11.7369) (27.5273, -10.9794) (27.5273, -10.2144) knots 0 0 0 1 2 2 2
  spline S93 degree 2 poles (28.1432, -10.2144) (28.1432, -10.7533) (28.3593, -11.2426) (28.5977, -11.2426) knots 0 0 0 1 2 2 2
  spline S94 degree 2 poles (28.5977, -11.2426) (28.8362, -11.2426) (29.0547, -10.7509) (29.0547, -10.2144) knots 0 0 0 1 2 2 2
  spline S95 degree 2 poles (29.0547, -10.2144) (29.0547, -9.6754) (28.8362, -9.1861) (28.5977, -9.1861) knots 0 0 0 1 2 2 2
  spline S96 degree 2 poles (28.5977, -9.1861) (28.3593, -9.1861) (28.1432, -9.6729) (28.1432, -10.2144) knots 0 0 0 1 2 2 2
  spline S97 degree 2 poles (29.934, -10.2144) (29.934, -9.4494) (30.4655, -8.6894) (31.0045, -8.6894) knots 0 0 0 1 2 2 2
  spline S98 degree 2 poles (31.0045, -8.6894) (31.5409, -8.6894) (32.0774, -9.4544) (32.0774, -10.2193) knots 0 0 0 1 2 2 2
  spline S99 degree 2 poles (32.0774, -10.2193) (32.0774, -10.9818) (31.5459, -11.7369) (31.0045, -11.7369) knots 0 0 0 1 2 2 2
  spline S100 degree 2 poles (31.0045, -11.7369) (30.4655, -11.7369) (29.934, -10.9794) (29.934, -10.2144) knots 0 0 0 1 2 2 2
  spline S101 degree 2 poles (30.5499, -10.2144) (30.5499, -10.7533) (30.766, -11.2426) (31.0045, -11.2426) knots 0 0 0 1 2 2 2
  spline S102 degree 2 poles (31.0045, -11.2426) (31.2429, -11.2426) (31.4615, -10.7509) (31.4615, -10.2144) knots 0 0 0 1 2 2 2
  spline S103 degree 2 poles (31.4615, -10.2144) (31.4615, -9.6754) (31.2429, -9.1861) (31.0045, -9.1861) knots 0 0 0 1 2 2 2
  spline S104 degree 2 poles (31.0045, -9.1861) (30.766, -9.1861) (30.5499, -9.6729) (30.5499, -10.2144) knots 0 0 0 1 2 2 2
  spline S105 degree 2 poles (32.3407, -10.2144) (32.3407, -9.4494) (32.8722, -8.6894) (33.4112, -8.6894) knots 0 0 0 1 2 2 2
  spline S106 degree 2 poles (33.4112, -8.6894) (33.9477, -8.6894) (34.4841, -9.4544) (34.4841, -10.2193) knots 0 0 0 1 2 2 2
  spline S107 degree 2 poles (34.4841, -10.2193) (34.4841, -10.9818) (33.9526, -11.7369) (33.4112, -11.7369) knots 0 0 0 1 2 2 2
  spline S108 degree 2 poles (33.4112, -11.7369) (32.8722, -11.7369) (32.3407, -10.9794) (32.3407, -10.2144) knots 0 0 0 1 2 2 2
  spline S109 degree 2 poles (32.9567, -10.2144) (32.9567, -10.7533) (33.1727, -11.2426) (33.4112, -11.2426) knots 0 0 0 1 2 2 2
  spline S110 degree 2 poles (33.4112, -11.2426) (33.6496, -11.2426) (33.8682, -10.7509) (33.8682, -10.2144) knots 0 0 0 1 2 2 2
  spline S111 degree 2 poles (33.8682, -10.2144) (33.8682, -9.6754) (33.6496, -9.1861) (33.4112, -9.1861) knots 0 0 0 1 2 2 2
  spline S112 degree 2 poles (33.4112, -9.1861) (33.1727, -9.1861) (32.9567, -9.6729) (32.9567, -10.2144) knots 0 0 0 1 2 2 2
  spline S113 degree 2 poles (34.7151, -11.6549) (34.7201, -11.2575) (35.0504, -10.7037) (35.4727, -10.4205) knots 0 0 0 1 2 2 2
  spline S114 degree 2 poles (35.4727, -10.4205) (35.5372, -10.3758) (35.6589, -10.3013) knots 0 0 0 1 1 1
  spline S115 degree 2 poles (35.6589, -10.3013) (36.2178, -9.9412) (36.2178, -9.6108) knots 0 0 0 1 1 1
  spline S116 degree 2 poles (36.2178, -9.6108) (36.2178, -9.4146) (35.9818, -9.1861) (35.7782, -9.1861) knots 0 0 0 1 2 2 2
  spline S117 degree 2 poles (35.7782, -9.1861) (35.5546, -9.1861) (35.3112, -9.4668) (35.3112, -9.7251) knots 0 0 0 1 2 2 2
  line L169 (35.3112, -9.7251) -> (35.3112, -9.7499)
  line L170 (35.3112, -9.7499) -> (34.7648, -9.7499)
  spline S118 degree 2 poles (34.7648, -9.7499) (34.7648, -9.2408) (35.3112, -8.6894) (35.8179, -8.6894) knots 0 0 0 1 2 2 2
  spline S119 degree 2 poles (35.8179, -8.6894) (36.2749, -8.6894) (36.8213, -9.1886) (36.8213, -9.6009) knots 0 0 0 1 2 2 2
  spline S120 degree 2 poles (36.8213, -9.6009) (36.8213, -9.8989) (36.5357, -10.3336) (36.1259, -10.6093) knots 0 0 0 1 2 2 2
  spline S121 degree 2 poles (36.1259, -10.6093) (36.0389, -10.6689) (35.885, -10.7682) knots 0 0 0 1 1 1
  spline S122 degree 2 poles (35.885, -10.7682) (35.495, -11.0166) (35.4453, -11.1483) knots 0 0 0 1 1 1
  line L171 (35.4453, -11.1483) -> (36.7915, -11.1483)
  line L172 (36.7915, -11.1483) -> (36.7915, -11.6549)
  line L173 (36.7915, -11.6549) -> (34.7151, -11.6549)
  line L174 (37.1492, -10.8105) -> (37.1492, -10.2417)
  line L175 (37.1492, -10.2417) -> (38.314, -10.2417)
  line L176 (38.314, -10.2417) -> (38.314, -10.8105)
  line L177 (38.314, -10.8105) -> (37.1492, -10.8105)
  spline S123 degree 2 poles (38.5723, -10.2144) (38.5723, -9.4494) (39.1038, -8.6894) (39.6428, -8.6894) knots 0 0 0 1 2 2 2
  spline S124 degree 2 poles (39.6428, -8.6894) (40.1793, -8.6894) (40.7158, -9.4544) (40.7158, -10.2193) knots 0 0 0 1 2 2 2
  spline S125 degree 2 poles (40.7158, -10.2193) (40.7158, -10.9818) (40.1843, -11.7369) (39.6428, -11.7369) knots 0 0 0 1 2 2 2
  spline S126 degree 2 poles (39.6428, -11.7369) (39.1038, -11.7369) (38.5723, -10.9794) (38.5723, -10.2144) knots 0 0 0 1 2 2 2
  spline S127 degree 2 poles (39.1883, -10.2144) (39.1883, -10.7533) (39.4044, -11.2426) (39.6428, -11.2426) knots 0 0 0 1 2 2 2
  spline S128 degree 2 poles (39.6428, -11.2426) (39.8813, -11.2426) (40.0998, -10.7509) (40.0998, -10.2144) knots 0 0 0 1 2 2 2
  spline S129 degree 2 poles (40.0998, -10.2144) (40.0998, -9.6754) (39.8813, -9.1861) (39.6428, -9.1861) knots 0 0 0 1 2 2 2
  spline S130 degree 2 poles (39.6428, -9.1861) (39.4044, -9.1861) (39.1883, -9.6729) (39.1883, -10.2144) knots 0 0 0 1 2 2 2
  line L178 (41.8906, -11.6549) -> (41.8906, -9.6282)
  line L179 (41.8906, -9.6282) -> (41.1827, -9.6282)
  line L180 (41.1827, -9.6282) -> (41.1827, -9.211)
  line L181 (41.1827, -9.211) -> (41.2274, -9.211)
  spline S131 degree 2 poles (41.2274, -9.211) (41.6149, -9.211) (41.9701, -8.97) (41.9999, -8.6894) knots 0 0 0 1 2 2 2
  line L182 (41.9999, -8.6894) -> (42.4742, -8.6894)
  line L183 (42.4742, -8.6894) -> (42.4742, -11.6549)
  line L184 (42.4742, -11.6549) -> (41.8906, -11.6549)
  line L185 (43.3808, -10.8105) -> (43.3808, -10.2417)
  line L186 (43.3808, -10.2417) -> (44.5457, -10.2417)
  line L187 (44.5457, -10.2417) -> (44.5457, -10.8105)
  line L188 (44.5457, -10.8105) -> (43.3808, -10.8105)
  line L189 (45.7577, -8.6049) -> (46.483, -8.6049)
  line L190 (46.483, -8.6049) -> (47.5832, -11.6549)
  line L191 (47.5832, -11.6549) -> (46.9251, -11.6549)
  line L192 (46.9251, -11.6549) -> (46.7164, -11.0266)
  line L193 (46.7164, -11.0266) -> (45.5342, -11.0266)
  line L194 (45.5342, -11.0266) -> (45.333, -11.6549)
  line L195 (45.333, -11.6549) -> (44.6723, -11.6549)
  line L196 (44.6723, -11.6549) -> (45.7577, -8.6049)
  line L197 (46.1228, -9.2159) -> (45.7006, -10.5124)
  line L198 (45.7006, -10.5124) -> (46.5475, -10.5124)
  line L199 (46.5475, -10.5124) -> (46.1228, -9.2159)
  point P0 (63.0835, -36.5)
  constraints: 2 other
emboss "Emboss1" sketch "Sketch6" operation add depth 0.5 direction (0, 0, -1)
equation "\"d5\" = box_length_outer"
equation "\"d6\" = box_width_outer"
equation "\"d23\" = wall_thickness"
equation "\"wall_thickness\" = 3"
equation "\"box_length_outer\" = box_length + 2 * wall_thickness"
equation "\"box_width_outer\" = 81"
equation "\"lid_screw_d\" = 4"
equation "\"min_wall_width\" = 1"
equation "\"box_width\" = 75"
equation "\"box_length\" = 150"
body "Solid1"
